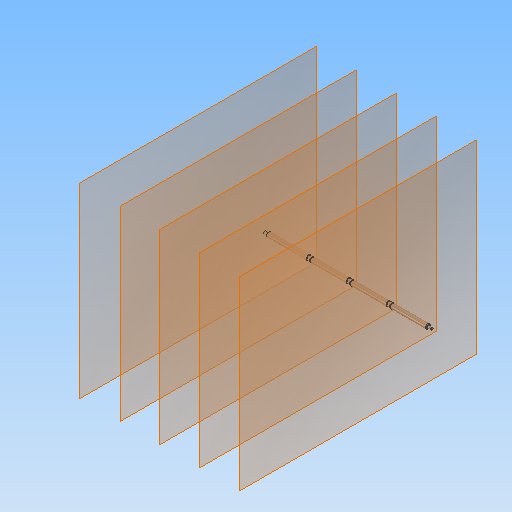
# Autodesk Inventor part: Timing_Lever Shaft 3 Lanes
Saved by Autodesk Inventor 2018.1 (Build 221171000, 171)
## iProperties
Created: 2019-02-07
Part Number: Timing_Lever Shaft 3 Lanes
Material: Steel, Mild
Document SubType Name: Modeling
Designer: James
Density: 7.85 g/cm^3
Appearance: Semi-Polished
Mass: 44.7989 g
Surface Area: 39.2758 cm^2
Volume: 5.70686 cm^3
Author: James
Autodesk Inventor part; units mm, degrees
ref_plane "YZ Plane" through (0, 0, 0) normal (1, 0, 0) x (0, 1, 0)
ref_plane "XZ Plane" through (0, 0, 0) normal (0, 1, 0) x (-1, 0, 0)
derived "Selection_Skeleton.ipt"
ref_plane "Ground" through (0, 0, 0) normal (0, 1, 0) x (-1, 0, 0)
ref_plane "LHS inner" through (0, 0, 0) normal (1, 0, 0) x (0, 1, 0)
ref_plane "RHS inner" through (300, 0, 0) normal (1, 0, 0) x (0, 1, 0)
ref_plane "Lane 1" through (50, 0, 0) normal (1, 0, 0) x (0, 1, 0)
ref_plane "Lane 2" through (100, 0, 0) normal (1, 0, 0) x (0, 1, 0)
ref_plane "Lane 3" through (150, 0, 0) normal (1, 0, 0) x (0, 1, 0)
ref_plane "Lane 4" through (200, 0, 0) normal (1, 0, 0) x (0, 1, 0)
ref_plane "Lane 5" through (250, 0, 0) normal (1, 0, 0) x (0, 1, 0)
ref_plane "Back" through (0, 0, 0) normal (0, 0, 1) x (1, 0, 0)
sketch "Sketch1" plane through (0, 0, 0) normal (1, 0, 0) x (0, 1, 0)
  circle A0 centre (0, 0) radius 3
  dimension "d1" = 6
  constraints: 1 centre point, 1 coincident
  measures "d1" diameter of A0
extrude "Extrusion1" add sketch "Sketch1" along normal up to surface (200 mm away)
sketch "Sketch2" plane through (200, 0, 0) normal (1, 0, 0) x (0, 0, -1)
  circle A0 centre (0, 0) radius 3 projected
extrude "Extrusion2" add sketch "Sketch2" along normal blind 5
sketch "Sketch3" plane through (0, 0, 0) normal (-1, 0, 0) x (0, 0, 1)
  circle A0 centre (0, 0) radius 3 projected
extrude "Extrusion3" add sketch "Sketch3" along normal blind 5
sketch "Sketch4" plane through (0, 0, 0) normal (0, 0, 1) x (1, 0, 0)
  line L0 (51, 3) -> (50.2, 3)
  line L1 (50.2, 3) -> (50.2, 2.85)
  line L2 (50.2, 2.85) -> (51, 2.85)
  line L3 (51, 2.85) -> (51, 3)
  line L4 (55.3, 3) -> (54.5, 3)
  line L5 (54.5, 3) -> (54.5, 2.85)
  line L6 (54.5, 2.85) -> (55.3, 2.85)
  line L7 (55.3, 2.85) -> (55.3, 3)
  line L8 (-17.06, 0) -> (67.36, 0) projected
  line L9 (-5, 3) -> (-5, -3) projected
  line L10 (50, 4.2) -> (50, -4.2) projected
  point P0 (0, 0)
  dimension "d8" = 2.85
  dimension "d9" = 0.8
  dimension "d10" = 0.8
  dimension "d11" = 3.5
  dimension "d13" = 1
  constraints: 16 end point, 4 parallel, 3 horizontal alignment, 2 horizontal, 2 perpendicular, 2 point on line
  measures "d8" distance between parallel lines of L8 L2
  measures "d9" distance of L0.start L0.end
  measures "d10" distance of L4.start L4.end
  measures "d11" distance between parallel lines of L3 L5
  measures "d13" distance from line of L10 L0.start
revolve "Revolution1" cut sketch "Sketch4" angle 360 about axis through (-10, 0, 0) along (1, 0, 0)
pattern_linear "Rectangular Pattern1" count 3 spacing 50 along (1, 0, 0) of "Revolution1"
sketch "Sketch5" plane through (0, 0, 0) normal (0, 0, 1) x (1, 0, 0)
  line L0 (-5, 3) -> (0, 3)
  line L1 (0, 3) -> (0, 1.5)
  line L2 (0, 1.5) -> (-5, 1.5)
  line L3 (-5, 1.5) -> (-5, 3)
  line L4 (-5, 3) -> (-5, -3) projected
  line L5 (-6, 0) -> (1, 0) projected
  point P0 (0, 0)
  dimension "d21" = 1.5
  dimension "d22" = 5
  constraints: 8 end point, 2 coincident, 2 parallel, 1 horizontal, 1 perpendicular
  measures "d21" distance between parallel lines of L5 L2
  measures "d22" distance of L0.start L0.end
revolve "Revolution2" cut sketch "Sketch5" angle 360 about axis through (-10, 0, 0) along (1, 0, 0)
ref_plane "mid plane" through (100, 0, 0) normal (-1, 0, 0) x (0, 0, 1)
mirror "Mirror1" about plane through (100, 0, 0) normal (-1, 0, 0) of "Revolution2"
chamfer "Chamfer2" distance 0.5 angle 45 2 edges at (-5, -1.5, 0) (205, -1.5, 0)
fillet "Fillet1" radius 0.5 2 edges at (200, -1.5, 0) (0, -1.5, 0)
chamfer "Chamfer3" distance 0.5 angle 45 2 edges at (0, 0, -3) (200, 0, -3)
equation "\"d10\" = d9"
body "Solid1"
